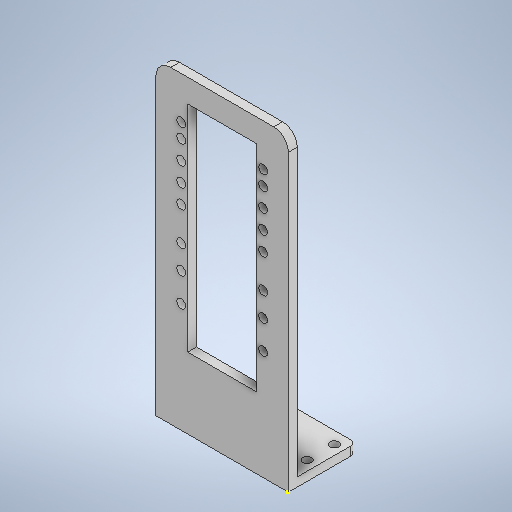
# Autodesk Inventor part: servo atach
Saved by Autodesk Inventor 2025.1 (Build 291241020, 241B)
## iProperties
Created: 2025-01-20
Part Number: servo atach
Material: Generic
Document SubType Name: Modeling
Designer: User
Density: 1 g/cm^3
Appearance: Default
Author: User
Autodesk Inventor part; units mm, degrees
ref_plane "YZ Plane" through (0, 0, 0) normal (1, 0, 0) x (0, 1, 0)
ref_plane "XZ Plane" through (0, 0, 0) normal (0, 1, 0) x (-1, 0, 0)
ref_plane "XY Plane" through (0, 0, 0) normal (0, 0, 1) x (1, 0, 0)
sketch "Sketch1" plane through (0, 0, 0) normal (0, 1, 0) x (-1, 0, 0)
  line L0 (0, 0) -> (45, 0)
  line L1 (45, 0) -> (45, -20)
  line L2 (45, -20) -> (0, -20)
  line L3 (0, -20) -> (0, 0)
  circle A0 centre (39.9418, -5.8805) radius 1.5
  circle A1 centre (39.4697, -15.8219) radius 1.5
  circle A2 centre (3.2694, -6.6358) radius 1.5
  circle A3 centre (3.2694, -15.8219) radius 1.5
  dimension "d0" = 45
  dimension "d1" = 20
  dimension "d4" = 3
  dimension "d5" = 3
  dimension "d6" = 3
  dimension "d7" = 3
  constraints: 8 end point, 4 centre point, 2 parallel, 1 horizontal, 1 perpendicular
  measures "d0" distance of L1.end L2.end
  measures "d1" distance of L0.end L1.end
  measures "d4" diameter of A0
  measures "d5" diameter of A1
  measures "d6" diameter of A2
  measures "d7" diameter of A3
extrude "Extrusion1" add sketch "Sketch1" along normal blind 3 contours L0 L1 L2 L3 | A0 | A1 | A2 | A3
extrude "Extrusion2" cut sketch "Sketch1" along normal through all contours A0 | A1 | A2 | A3
sketch "Sketch2" plane through (-45, 0, 0) normal (0, 0, 1) x (1, 0, 0)
  line L0 (0, 0) -> (45, 0)
  line L1 (45, 0) -> (45, 105)
  line L2 (45, 105) -> (0, 105)
  line L3 (0, 105) -> (0, 0)
  line L4 (10.782, 97.156) -> (34.218, 97.156)
  line L5 (34.218, 97.156) -> (34.218, 84.256)
  line L6 (34.218, 84.256) -> (10.782, 84.256)
  line L7 (10.782, 84.256) -> (10.782, 97.156)
  circle A0 centre (8.582, 90.706) radius 1.5
  circle A1 centre (36.418, 90.706) radius 1.5
  line L8 (10.782, 79.3472) -> (34.218, 79.3472)
  line L9 (34.218, 79.3472) -> (34.218, 66.4472)
  line L10 (34.218, 66.4472) -> (10.782, 66.4472)
  line L11 (10.782, 66.4472) -> (10.782, 79.3472)
  circle A2 centre (8.582, 72.8972) radius 1.5
  circle A3 centre (36.418, 72.8972) radius 1.5
  line L12 (10.782, 61.5315) -> (34.218, 61.5315)
  line L13 (34.218, 61.5315) -> (34.218, 48.6315)
  line L14 (34.218, 48.6315) -> (10.782, 48.6315)
  line L15 (10.782, 48.6315) -> (10.782, 61.5315)
  circle A4 centre (8.582, 55.0815) radius 1.5
  circle A5 centre (36.418, 55.0815) radius 1.5
  circle A6 centre (36.418, 37.2658) radius 1.5
  circle A7 centre (8.582, 37.2658) radius 1.5
  line L16 (10.782, 30.8158) -> (10.782, 43.7158)
  line L17 (34.218, 30.8158) -> (10.782, 30.8158)
  line L18 (34.218, 43.7158) -> (34.218, 30.8158)
  line L19 (10.782, 43.7158) -> (34.218, 43.7158)
  line L20 (10.782, 97.156) -> (34.218, 97.156)
  line L21 (34.218, 97.156) -> (34.218, 24.1177)
  line L22 (34.218, 24.1177) -> (10.782, 24.1177)
  line L23 (10.782, 24.1177) -> (10.782, 97.156)
  circle A8 centre (8.582, 85.7719) radius 1.5
  circle A9 centre (36.418, 85.7719) radius 1.5
  circle A10 centre (8.582, 79.3472) radius 1.5
  circle A11 centre (36.418, 79.3472) radius 1.5
  circle A12 centre (8.582, 66.4472) radius 1.5
  circle A13 centre (36.418, 66.4472) radius 1.5
  circle A14 centre (36.418, 46.9762) radius 1.5
  circle A15 centre (8.582, 46.9762) radius 1.5
  point P0 (10.782, 90.706)
  point P1 (10.782, 72.8972)
  point P2 (10.782, 55.0815)
  point P3 (10.782, 37.2658)
  dimension "d10" = 105
  dimension "d13" = 45
  dimension "d14" = 23.436
  dimension "d15" = 12.9
  dimension "d17" = 10.782
  dimension "d18" = 3
  dimension "d19" = 3
  dimension "d20" = 2.2
  dimension "d21" = 2.2
  dimension "d22" = 23.436
  dimension "d23" = 12.9
  dimension "d24" = 3
  dimension "d25" = 3
  dimension "d26" = 2.2
  dimension "d27" = 2.2
  dimension "d28" = 23.436
  dimension "d29" = 12.9
  dimension "d30" = 3
  dimension "d31" = 3
  dimension "d32" = 2.2
  dimension "d33" = 2.2
  dimension "d34" = 23.436
  dimension "d35" = 12.9
  dimension "d36" = 3
  dimension "d37" = 3
  dimension "d38" = 2.2
  dimension "d39" = 2.2
  dimension "d44" = 3
  dimension "d45" = 3
  dimension "d46" = 3
  dimension "d47" = 3
  dimension "d48" = 3
  dimension "d49" = 3
  dimension "d50" = 3
  dimension "d51" = 3
  constraints: 48 end point, 16 centre point, 12 parallel, 6 horizontal, 6 perpendicular, 4 midpoint, 1 point on line
  measures "d10" distance of L0.end L1.end
  measures "d13" distance of L1.end L2.end
  measures "d14" distance of L5.end L6.end
  measures "d15" distance of L4.end L5.end
  measures "d17" distance between parallel lines of L3 L7
  measures "d18" diameter of A0
  measures "d19" diameter of A1
  measures "d20" distance from line of A1.centre L5
  measures "d21" distance of point (10.782, 90.706) A0.centre
  measures "d22" distance of L10.start L11.start
  measures "d23" distance of L9.start L10.start
  measures "d24" diameter of A2
  measures "d25" diameter of A3
  measures "d26" distance from line of A3.centre L9
  measures "d27" distance of point (10.782, 72.897) A2.centre
  measures "d28" distance of L14.start L15.start
  measures "d29" distance of L13.start L14.start
  measures "d30" diameter of A4
  measures "d31" diameter of A5
  measures "d32" distance from line of A5.centre L13
  measures "d33" distance of point (10.782, 55.082) A4.centre
  measures "d34" distance of L18.end L17.end
  measures "d35" distance of L19.end L18.end
  measures "d36" diameter of A7
  measures "d37" diameter of A6
  measures "d38" distance from line of A6.centre L18
  measures "d39" distance of point (10.782, 37.266) A7.centre
  measures "d44" diameter of A8
  measures "d45" diameter of A9
  measures "d46" diameter of A10
  measures "d47" diameter of A11
  measures "d48" diameter of A12
  measures "d49" diameter of A13
  measures "d50" diameter of A15
  measures "d51" diameter of A14
extrude "Extrusion3" add sketch "Sketch2" along normal blind 3 contours L3 L2 L1 L0 | L4 L5 L6 L7 | L6 L21 L8 L23 | L8 L9 L10 L11 | L10 L21 L12 L23 | L12 L13 L14 L15 | L14 L21 L19 L23 | L19 L18 L17 L16 | L17 L21 L22 L23 | A0 | A1 | A2 | A3 | A4 | A5 | A6 | A7 | A8 | A9 | A10 | A11 | A12 | A13 | A14 | A15
extrude "Extrusion4" cut sketch "Sketch2" along normal through all contours L4 L5 L6 L7 | L8 L9 L10 L11 | L12 L13 L14 L15 | L19 L18 L17 L16 | A0 | A1 | A2 | A3 | A4 | A5 | A6 | A7
extrude "Extrusion5" cut sketch "Sketch2" along normal through all contours L6 L21 L8 L23 | L10 L21 L12 L23 | L14 L21 L19 L23 | L17 L21 L22 L23
extrude "Extrusion6" cut sketch "Sketch2" along normal blind 3 contours A8 | A9 | A10 | A11 | A12 | A13 | A14 | A15
fillet "Fillet1" radius 5 1 edges at (-45, 105, 1.5)
fillet "Fillet2" radius 5 1 edges at (0, 105, 1.5)
fillet "Fillet3" radius 2 2 edges at (0, 1.5, -20) (-45, 1.5, -20)
sketch "Sketch4" plane through (-45, 0, 3) normal (0, 0, 1) x (1, 0, 0)
  point P0 (45, 0)
equation "\"d52\" = d48"
body "Solid1"
